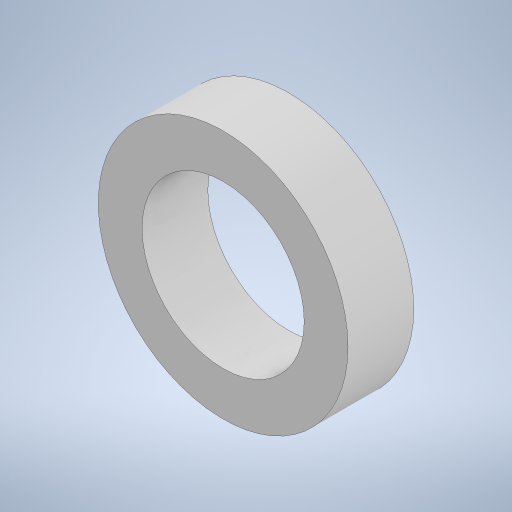
# Autodesk Inventor part: back
Saved by Autodesk Inventor 2023 (Build 270158000, 158)
## iProperties
Created: 2022-09-21
Part Number: back
Material: Generic
Document SubType Name: Modeling
Designer: station
Density: 1 g/cm^3
Appearance: Default
Author: station
Autodesk Inventor part; units mm, degrees
ref_plane "YZ Plane" through (0, 0, 0) normal (1, 0, 0) x (0, 1, 0)
ref_plane "XZ Plane" through (0, 0, 0) normal (0, 1, 0) x (-1, 0, 0)
ref_plane "XY Plane" through (0, 0, 0) normal (0, 0, 1) x (1, 0, 0)
sketch "Sketch1" plane through (0, 0, 0) normal (0, 0, 1) x (1, 0, 0)
  circle A0 centre (0, 0) radius 18.5
  circle A1 centre (0, 0) radius 28.5
  circle A2 centre (0, 0) radius 23.5 construction
  circle A3 centre (0, 23.5) radius 3 construction
  circle A4 centre (0, 0) radius 26.5
  dimension "d5" = 47
  dimension "d0" = 37
  dimension "d1" = 57
  dimension "d6" = 6
  dimension "d11" = 53
  constraints: 4 centre point, 4 coincident, 1 vertical alignment, 2 other
  measures "d0" diameter of A0
  measures "d1" diameter of A1
  measures "d6" diameter of A3
  measures "d11" diameter of A4
extrude "Extrusion1" add sketch "Sketch1" along normal blind 15 contours A1 | A4
body "Solid1"
